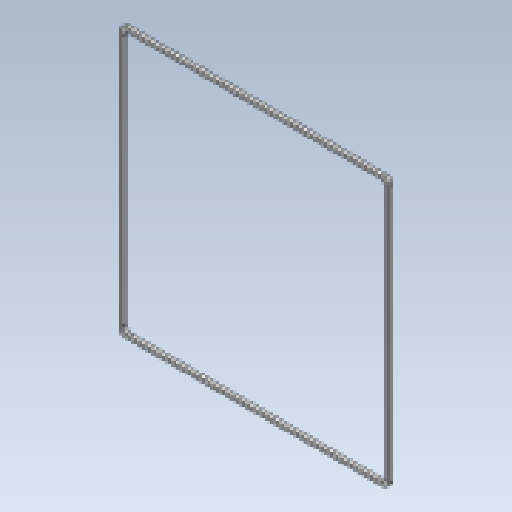
# Autodesk Inventor part: border
Saved by Autodesk Inventor 2023 (Build 270158030, 158C)
## iProperties
Created: 2024-12-24
Part Number: border
Material: Generic
Document SubType Name: Modeling
Designer: Imogen Heard
Density: 1 g/cm^3
Appearance: Default
Author: Imogen Heard
Autodesk Inventor part; units mm, degrees
ref_plane "YZ Plane" through (0, 0, 0) normal (1, 0, 0) x (0, 1, 0)
ref_plane "XZ Plane" through (0, 0, 0) normal (0, 1, 0) x (-1, 0, 0)
ref_plane "XY Plane" through (0, 0, 0) normal (0, 0, 1) x (1, 0, 0)
sketch "Sketch1" plane through (0, 0, 0) normal (0, 0, 1) x (1, 0, 0)
  line L0 (-115, 115) -> (115, 115)
  line L1 (115, 115) -> (115, -115)
  line L2 (115, -115) -> (-115, -115)
  line L3 (-115, -115) -> (-115, 115)
  line L4 (112, 112) -> (-112, 112)
  line L5 (-112, 112) -> (-112, -112)
  line L6 (-112, -112) -> (112, -112)
  line L7 (112, -112) -> (112, 112)
  point P0 (0, 0)
  dimension "d0" = 230
  dimension "d1" = 230
  dimension "d2" = 115
  dimension "d3" = 115
  dimension "d4" = 3
  constraints: 16 end point, 4 parallel, 2 perpendicular, 1 horizontal, 3 other
  measures "d0" distance between parallel lines of L1 L3
  measures "d1" distance between parallel lines of L2 L0
  measures "d2" distance from line of point (0, 0) L0
  measures "d3" distance from line of L3 point (0, 0)
  measures "d4" distance between parallel lines of L5 L3
extrude "Extrusion1" add sketch "Sketch1" against normal blind 3
fillet "Fillet1" radius 5 8 edges at (-115, 115, -1.5) (-112, 112, -1.5) (-112, -112, -1.5) (-115, -115, -1.5) (115, -115, -1.5) (112, -112, -1.5) (115, 115, -1.5) (112, 112, -1.5)
equation "\"d1\" = d0"
equation "\"d2\" = 0.5 * d0"
equation "\"d3\" = 0.5 * d0"
body "Solid1"
